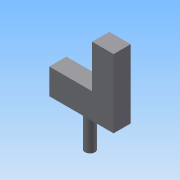
# Autodesk Inventor part: tete_bras
Saved by Autodesk Inventor 2013 (Build 170138000, 138)
## iProperties
Created: 2012-11-14
Part Number: tete_bras
Material: Générique
Document SubType Name: Modeling
Designer: Aegir
Density: 1 g/cm^3
Author: Aegir
Autodesk Inventor part; units mm, degrees
ref_plane "YZ Plane" through (0, 0, 0) normal (1, 0, 0) x (0, 1, 0)
ref_plane "XZ Plane" through (0, 0, 0) normal (0, 1, 0) x (-1, 0, 0)
ref_plane "XY Plane" through (0, 0, 0) normal (0, 0, 1) x (1, 0, 0)
sketch "Esquisse1" plane through (0, 0, 0) normal (0, 1, 0) x (-1, 0, 0)
  line L0 (0, 0) -> (-150, 0)
  line L1 (-150, 0) -> (-150, 63.6055)
  line L2 (-100, 60) -> (0, 60)
  line L3 (0, 60) -> (0, 0)
  line L4 (-100, 60) -> (-100, 160)
  line L5 (-100, 160) -> (-150, 160)
  line L6 (-150, 160) -> (-150, 63.6055)
  dimension "d2" = 100
  dimension "d4" = 60
  dimension "d5" = 100
  dimension "d6" = 150
  constraints: 14 end point, 3 parallel, 1 horizontal, 1 perpendicular
  measures "d2" distance of L2.start L4.end
  measures "d4" distance between parallel lines of L0 L2
  measures "d5" distance of L2.start L2.end
  measures "d6" distance between parallel lines of L3 L1
extrude "Extrusion1" add sketch "Esquisse1" along normal blind 40
sketch "Esquisse2" plane through (150, 0, 0) normal (0, 0, -1) x (-1, 0, 0)
  circle A0 centre (75, 20) radius 11.5999
  constraints: 1 centre point
extrude "Extrusion2" add sketch "Esquisse2" along normal blind 80
